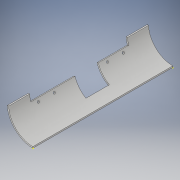
# Autodesk Inventor part: lowerClaw
Saved by Autodesk Inventor 2017 (Build 210142000, 142)
## iProperties
Created: 2017-04-06
Part Number: lowerClaw
Material: Generic
Document SubType Name: Modeling
Designer: s4461999
Density: 1 g/cm^3
Appearance: Default
Author: s4461999
Autodesk Inventor part; units mm, degrees
ref_plane "YZ Plane" through (0, 0, 0) normal (1, 0, 0) x (0, 1, 0)
ref_plane "XZ Plane" through (0, 0, 0) normal (0, 1, 0) x (-1, 0, 0)
ref_plane "XY Plane" through (0, 0, 0) normal (0, 0, 1) x (1, 0, 0)
sketch "Sketch1" plane through (0, 0, 0) normal (0, 0, 1) x (1, 0, 0)
  line L0 (0, 0) -> (0, 3)
  arc A0 (-49.4773, 39) -> (0, 3) centre (0, 55) ccw
  line L1 (-49.4773, 39) -> (-52.3317, 38.0769)
  arc A1 (-52.3317, 38.0769) -> (0, 0) centre (0, 55) ccw
  dimension "d0" = 55
  dimension "d1" = 52
  dimension "d4" = 36
  dimension "d5" = 39
  dimension "d6" = 0
  dimension "d7" = 0
  constraints: 4 end point, 4 point on circle, 2 centre point, 1 line through centre, 1 vertical
  measures "d0" radius of A1
  measures "d1" radius of A0
  measures "d4" vertical distance of L0.end L1.start
  measures "d5" vertical distance of L0.start L1.start
  measures "d6" distance of A1.centre A0.centre
  measures "d7" distance from line of L0 A1.centre
extrude "Extrusion1" add sketch "Sketch1" along normal blind 300
sketch "Sketch4" plane through (0, 0, 300) normal (0, 0, 1) x (1, 0, 0)
  point P0 (0, 0)
sketch "Sketch5" plane through (0, 0, 0) normal (0, 0, -1) x (-1, 0, 0)
  arc A0 (0, 3) -> (49.4773, 39) centre (0, 55) ccw projected
  line L0 (0, 55) -> (49.8792, 31.8254)
  line L1 (49.4773, 39) -> (52.3317, 38.0769) projected
  point P0 (0, 0)
  dimension "d27" = 7
  dimension "d28" = 55
  constraints: 2 end point
  measures "d27" angle of L0 L1
  measures "d28" distance of L0.start L0.end
ref_plane "Work Plane3" through (-49.8792, 31.8254, 0) normal (-0.9068954, -0.4213558, 0) x (0.4213558, -0.9068954, 0)
sketch "Sketch6" plane through (0, 0, 0) normal (0, 0, -1) x (-1, 0, 0)
  point P0 (0, 0)
sketch "Sketch7" plane through (-49.8792, 31.8254, 0) normal (-0.9068954, -0.4213558, 0) x (0.4213558, -0.9068954, 0)
  point P0 (49.8792, 0)
sketch "Sketch8" plane through (-49.8792, 31.8254, 0) normal (-0.9068954, -0.4213558, 0) x (0.4213558, -0.9068954, 0)
  line L0 (49.8792, 0) -> (-6.7028, 0) projected
  line L1 (-54.9925, 150) -> (98.8882, 150)
  line L2 (-6.7028, 0) -> (-6.7028, 300) projected
  point P0 (0.0122, 59)
  point P1 (0.0122, 93)
  point P2 (0.0122, 241)
  point P3 (0.0122, 207)
  dimension "d30" = 150
  dimension "d31" = 57
  dimension "d32" = 34
  dimension "d33" = 6.715
  dimension "d34" = 6.715
  constraints: 2 end point, 2 symmetric about line, 1 horizontal
  measures "d30" distance between parallel lines of L0 L1
  measures "d31" distance from line of point (0.012, 93) L1
  measures "d32" distance of point (0.012, 93) point (0.012, 59)
  measures "d33" distance from line of L2 point (0.012, 59)
  measures "d34" distance from line of L2 point (0.012, 93)
hole "Hole2" at (-49.8741, 31.8144, 59) at (-49.8741, 31.8144, 93) at (-49.8741, 31.8144, 207) at (-49.8741, 31.8144, 241) direction (0.9068954, 0.4213558, 0) diameter 4.4 end through all
sketch "Sketch9" plane through (-49.8792, 31.8254, 0) normal (-0.9068954, -0.4213558, 0) x (0.4213558, -0.9068954, 0)
  line L0 (-54.3753, 150) -> (83.8771, 150)
  line L1 (49.8792, 0) -> (-6.7028, 0) projected
  line L2 (-11.8554, 110.2) -> (33, 110.2)
  line L3 (33, 110.2) -> (33, 160.2)
  line L4 (33, 160.2) -> (-11.8554, 160.2)
  line L5 (-11.8554, 160.2) -> (-11.8554, 110.2)
  point P0 (0, 95.2)
  dimension "d42" = 150
  dimension "d43" = 33
  dimension "d46" = 15
  dimension "d47" = 50
  constraints: 10 end point, 2 horizontal, 2 parallel, 1 perpendicular
  measures "d42" distance between parallel lines of L0 L1
  measures "d43" distance from line of L3 point (0, 95.2)
  measures "d46" distance from line of L2 point (0, 95.2)
  measures "d47" distance of L4.end L2.start
extrude "Extrusion2" cut sketch "Sketch9" against normal blind 10
ref_plane "Work Plane4" through (-27.4859, 7.3604, 0) normal (-0.4997428, -0.8661738, 0) x (0.8661738, -0.4997428, 0)
sketch "Sketch10" plane through (-27.4859, 7.3604, 0) normal (-0.4997428, -0.8661738, 0) x (0.8661738, -0.4997428, 0)
  line L0 (0, 110.2) -> (-4.5533, 110.2) projected
  line L1 (0, 160.2) -> (0, 110.2) projected
  line L2 (-4.5533, 110.2) -> (0, 110.2)
  line L3 (0, 110.2) -> (0, 160.2)
  line L4 (0, 160.2) -> (-4.5533, 160.2)
  line L5 (-4.5533, 160.2) -> (-4.5533, 110.2)
  point P0 (27.4859, 0)
  constraints: 8 end point, 2 parallel, 1 horizontal, 1 perpendicular
extrude "Extrusion3" cut sketch "Sketch10" against normal blind 10
sketch "Sketch11" plane through (0, 0, 0) normal (0, 0, -1) x (-1, 0, 0)
  line L0 (49.4773, 39) -> (52.3317, 38.0769) projected
  line L1 (49.4773, 39) -> (52.3317, 38.0769)
  arc A0 (49.4773, 39) -> (51.9325, 52.3508) centre (0, 55) ccw
  arc A1 (27.4859, 7.3604) -> (52.3317, 38.0769) centre (0, 55) ccw projected
  arc A2 (52.3317, 38.0769) -> (54.9286, 52.198) centre (0, 55) ccw
  line L2 (51.9325, 52.3508) -> (54.9286, 52.198)
  point P0 (0, 0)
  dimension "d52" = 52
  dimension "d53" = 55
  dimension "d54" = 15
  constraints: 4 end point, 4 point on circle, 2 centre point, 1 collinear, 1 concentric, 1 line through centre
  measures "d52" radius of A0
  measures "d53" radius of A2
  measures "d54" angle of L0 L2
extrude "Extrusion4" add sketch "Sketch11" against normal blind 45
ref_plane "Work Plane5" through (0, 0, 150) normal (0, 0, -1) x (-1, 0, 0)
mirror "Mirror1" about plane through (0, 0, 150) normal (0, 0, -1) of "Extrusion4"
body "Solid1"
